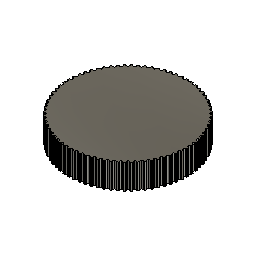
gear_76z (Autodesk Fusion 360 design; units mm, degrees)
Autodesk Fusion 360 part; units mm, degrees
sketch "Sketch1" plane through (0, 0, 0) normal (0, 0, 1) x (1, 0, 0) in component "gt2 pulley"
  circle A0 centre (0, 0) radius 24.1916 construction
  circle A1 centre (0, 0) radius 23.1876 construction
  line L0 (0, 0) -> (0, 24.1916) construction
  line L1 (0, 0) -> (0.9997, 24.1709) construction
  line L2 (0, 0) -> (1.4051, 24.1507) construction
  circle A2 centre (0, 0) radius 23.9376 construction
  arc A3 (0.395, 23.8007) -> (0.4708, 23.5042) centre (1.3904, 23.8971) ccw
  circle A4 centre (0, 0) radius 23.7876 construction
  arc A5 (0.2472, 23.9363) -> (0, 23.9376) centre (0, 0) ccw
  arc A6 (0.395, 23.8007) -> (0.2472, 23.9363) centre (0.2457, 23.7863) ccw
  arc A7 (0.4708, 23.5042) -> (0.9582, 23.1677) centre (0.9812, 23.7223) ccw
  arc A8 (0, 23.9376) -> (-0.2472, 23.9363) centre (0, 0) ccw
  arc A9 (-0.2472, 23.9363) -> (-0.395, 23.8007) centre (-0.2457, 23.7863) ccw
  arc A10 (-0.4708, 23.5042) -> (-0.395, 23.8007) centre (-1.3904, 23.8971) ccw
  arc A11 (-0.958, 23.1678) -> (-0.4708, 23.5042) centre (-0.9812, 23.7223) ccw
  arc A12 (0.9582, 23.1677) -> (-0.9582, 23.1677) centre (0, 0) ccw
  point P0 (1.3904, 23.8971)
  point P1 (0, 23.9376)
  dimension "d18" = 48.3831
  dimension "d19" = 2.368
  dimension "d22" = 1.004
  dimension "d24" = 0.75
  dimension "d26" = 1
  dimension "d27" = 0.15
  dimension "d28" = 0.15
  dimension "d47" = 0.555
  dimension "d52" = 3.812
  constraint coincident A0.centre A1.centre
  constraint coincident A0 L0.end
  constraint vertical L0
  constraint coincident A0 L1.end
  constraint coincident A0 L2.end
  constraint concentric A1 A2
  constraint coincident A1 A7.end
  constraint coincident L1 A7.end
  constraint coincident A2 P0
  constraint coincident L2 P0
  constraint coincident P0 A3.centre
  constraint coincident A2 P1
  constraint coincident L0 P1
  constraint concentric A2 A4
  constraint coincident P1 A5.end
  constraint coincident A4 A6.centre
  constraint coincident A3.start A6.start
  constraint tangent A3 A6
  constraint tangent A3 A7
  constraint symmetric L0 A7.end A12.end
  constraint symmetric L0 A3.start A9.end
  constraint symmetric L0 A3.end A10.start
  constraint symmetric L0 A3 A10
  constraint symmetric L0 A5.start A8.end
  constraint symmetric L0 P1 A5.end
  constraint symmetric L0 A5 A8
  constraint symmetric L0 A6 A9
  constraint symmetric L0 A7 A11
  constraint coincident A1 A11.start
  constraint tangent A1 A7
  constraint coincident L1 A7.centre
  measures "d18" diameter of A0
  measures "d19" angle of L0 L1
  measures "d22" distance of A0 A1
  measures "d24" distance of A1 A2
  measures "d26" radius of A3
  measures "d27" distance of A2 A4
  measures "d28" radius of A6
  measures "d47" radius of A7
extrude "Extrude1" add sketch "Sketch1" along normal blind 10 makes body 1
pattern_circular "C-Pattern1" count 76 over 360 about axis through (0, 0, 1.75) along (0, 0, 1) of bodies 1 makes body 2 at (-1.171, 23.158, 3.3333) makes body 3 at (-3.9214, 22.8536, 6.6667) makes body 4 at (-6.4117, 22.2835, 6.6667) makes body 5 at (-6.8201, 22.1619, 3.3333) makes body 6 at (-9.992, 20.9242, 6.6667) makes body 7 at (-10.3748, 20.7371, 3.3333) makes body 8 at (-13.2997, 18.9942, 6.6667) makes body 9 at (-14.3259, 18.2327, 6.6667) makes body 10 at (-16.2446, 16.5461, 6.6667) makes body 11 at (-16.546, 16.2448, 3.3333) makes body 12 at (-17.831, 14.8229, 3.3333) makes body 13 at (-19.4698, 12.5932, 6.6667) makes body 14 at (-20.737, 10.375, 6.6667) makes body 15 at (-20.9241, 9.9921, 3.3333) makes body 16 at (-22.1618, 6.8203, 6.6667) makes body 17 at (-22.2834, 6.4118, 3.3333) makes body 18 at (-22.7368, 4.5498, 3.3333) makes body 19 at (-23.1169, 1.8088, 6.6667) makes body 20 at (-23.1756, -0.7452, 6.6667) makes body 21 at (-23.158, -1.171, 3.3333) makes body 22 at (-22.8536, -3.9214, 6.6667) makes body 23 at (-22.6494, -4.9667, 3.3333) makes body 24 at (-21.6779, -8.2299, 6.6667) makes body 25 at (-21.523, -8.6269, 3.3333) makes body 26 at (-20.7371, -10.3748, 3.3333) makes body 27 at (-18.9942, -13.2997, 6.6667) makes body 28 at (-18.2327, -14.3259, 6.6667) makes body 29 at (-16.5461, -16.2446, 6.6667) makes body 30 at (-16.2448, -16.546, 3.3333) makes body 31 at (-14.8229, -17.831, 3.3333) makes body 32 at (-13.2999, -18.9941, 3.3333) makes body 33 at (-10.375, -20.737, 6.6667) makes body 34 at (-9.2168, -21.2771, 6.6667) makes body 35 at (-6.8203, -22.1618, 6.6667) makes body 36 at (-6.4118, -22.2834, 3.3333) makes body 37 at (-4.5498, -22.7368, 3.3333) makes body 38 at (-1.8088, -23.1169, 6.6667) makes body 39 at (0.7452, -23.1756, 6.6667) makes body 40 at (2.4448, -23.0583, 6.6667) makes body 41 at (3.9214, -22.8536, 6.6667) makes body 42 at (6.4117, -22.2835, 6.6667) makes body 43 at (6.8201, -22.1619, 3.3333) makes body 44 at (9.992, -20.9242, 6.6667) makes body 45 at (10.3748, -20.7371, 3.3333) makes body 46 at (12.0518, -19.8095, 3.3333) makes body 47 at (14.3259, -18.2327, 6.6667) makes body 48 at (15.148, -17.5557, 3.3333) makes body 49 at (16.546, -16.2448, 3.3333) makes body 50 at (17.831, -14.8229, 3.3333) makes body 51 at (18.9941, -13.2999, 6.6667) makes body 52 at (20.737, -10.375, 6.6667) makes body 53 at (20.9241, -9.9921, 3.3333) makes body 54 at (22.1618, -6.8203, 6.6667) makes body 55 at (22.2834, -6.4118, 3.3333) makes body 56 at (22.7368, -4.5498, 3.3333) makes body 57 at (23.158, -1.1712, 6.6667) makes body 58 at (23.1756, 0.7452, 6.6667) makes body 59 at (23.158, 1.171, 3.3333) makes body 60 at (22.8536, 3.9214, 6.6667) makes body 61 at (22.6494, 4.9667, 3.3333) makes body 62 at (21.6779, 8.2299, 6.6667) makes body 63 at (21.523, 8.6269, 3.3333) makes body 64 at (20.7371, 10.3748, 3.3333) makes body 65 at (19.8095, 12.0518, 3.3333) makes body 66 at (18.7466, 13.6465, 3.3333) makes body 67 at (16.9874, 15.7826, 6.6667) makes body 68 at (16.2448, 16.546, 3.3333) makes body 69 at (14.8229, 17.831, 3.3333) makes body 70 at (13.2999, 18.9941, 3.3333) makes body 71 at (10.375, 20.737, 6.6667) makes body 72 at (9.9921, 20.9241, 3.3333) makes body 73 at (6.8203, 22.1618, 6.6667) makes body 74 at (5.589, 22.5039, 6.6667) makes body 75 at (3.0795, 22.9821, 6.6667) makes body 76 at (2.6567, 23.0349, 3.3333)
sketch "Sketch2" plane through (0, 0, 10) normal (0, 0, 1) x (-1, 0, 0)
  arc A0 (-4.3071, -23.4111) -> (-4.1836, -23.5691) centre (-4.1575, -23.4214) ccw
  arc A1 (-4.1836, -23.5691) -> (-3.696, -23.6505) centre (0, 0) ccw
  arc A2 (-3.696, -23.6505) -> (-3.5278, -23.5411) centre (-3.6727, -23.5023) ccw
  arc A3 (-3.4043, -23.2611) -> (-3.5278, -23.5411) centre (-2.5619, -23.8001) ccw
  arc A4 (-2.8683, -23.0095) -> (-3.4043, -23.2611) centre (-2.9368, -23.5602) ccw
  arc A5 (-4.7584, -22.694) -> (-2.8683, -23.0095) centre (0, 0) ccw
  arc A6 (-4.333, -23.1061) -> (-4.7584, -22.694) centre (-4.8723, -23.2372) ccw
  arc A7 (-4.3071, -23.4111) -> (-4.333, -23.1061) centre (-5.3047, -23.3424) ccw
  circle A8 centre (0, 0) radius 23.1876
  constraint coincident A1.centre A5.centre
extrude "Extrude2" add sketch "Sketch2" against normal blind 10 contours A5 A8 bodies 1 2 3 4 5 6 7 8 9 10 11 12 13 14 15 16 17 18 19 20 21 22 23 24 25 26 27 28 29 30 31 32 33 34 35 36 37 38 39 40 41 42 43 44 45 46 47 48 49 50 51 52 53 54 55 56 57 58 59 60 61 62 63 64 65 66 67 68 69 70 71 72 73 74 75 76
extrude "Extrude4" [suppressed] in component "gt2 pulley"
pattern_circular "C-Pattern7" [suppressed] in component "gt2 pulley"
extrude "Extrude3" [suppressed] in component "gt2 pulley"
pattern_circular "C-Pattern6" [suppressed] in component "gt2 pulley"
extrude "Extrude2'" [suppressed] in component "gt2 pulley"
pattern_circular "C-Pattern5" [suppressed] in component "gt2 pulley"
extrude "Extrude1'" [suppressed] in component "gt2 pulley"
pattern_circular "C-Pattern4" [suppressed] in component "gt2 pulley"
pattern_circular "C-Pattern3" [suppressed] in component "gt2 pulley"
pattern_circular "C-Pattern2" [suppressed] in component "gt2 pulley"
pattern_circular "C-Pattern1'" [suppressed] in component "gt2 pulley"
copy_body "Body->Comp1" [suppressed] in component "Component"
copy_body "Body->Comp2" [suppressed] in component "Component'"
copy_body "Body->Comp3" [suppressed] in component "Component''"
copy_body "Body->Comp4" [suppressed] in component "Component'''"
copy_body "Body->Comp5" [suppressed] in component "Component''''"
copy_body "Body->Comp6" [suppressed] in component "Component'''''"
copy_body "Body->Comp7" [suppressed] in component "Component''''''"
copy_body "Body->Comp8" [suppressed] in component "Component'''''''"
copy_body "Body->Comp9" [suppressed] in component "Component''''''''"
copy_body "Body->Comp10" [suppressed] in component "Component'''''''''"
copy_body "Body->Comp11" [suppressed] in component "Component''''''''''"
copy_body "Body->Comp12" [suppressed] in component "Component'''''''''''"
copy_body "Body->Comp13" [suppressed] in component "Component''''''''''''"
copy_body "Body->Comp14" [suppressed] in component "Component'''''''''''''"
copy_body "Body->Comp15" [suppressed] in component "Component''''''''''''''"
copy_body "Body->Comp16" [suppressed] in component "Component'''''''''''''''"
copy_body "Body->Comp17" [suppressed] in component "Component''''''''''''''''"
copy_body "Body->Comp18" [suppressed] in component "Component'''''''''''''''''"
copy_body "Body->Comp19" [suppressed] in component "Component''''''''''''''''''"
copy_body "Body->Comp20" [suppressed] in component "Component'''''''''''''''''''"
component "gt2 pulley" placed x (1, 0, 0) y (0, 1, 0) z (0, 0, 1) at (0, 0, 0)
equation "NumTeeth = 76" comment "min 20"
equation "ToothPitch = 2 mm"
equation "PullyDia = NumTeeth * ToothPitch / PI"
equation "ToothAng = ( ( 360 / NumTeeth ) * 1 deg )"
equation "TransOffsetAngle = ToothAng * 0.2"
equation "Sholulder_Radius = 0.15 mm"
equation "Root_Radius = 0.555 mm"
equation "TransRadius = 1 mm"
equation "ToolHeight = 0.75 mm"
equation "PLD = 0.254 mm"
equation "d18 = PullyDia"
equation "d19 = ToothAng / 2"
equation "d22 = PLD + ToolHeight"
equation "d24 = ToolHeight"
equation "d26 = TransRadius"
equation "d27 = Sholulder_Radius"
equation "d31 = NumTeeth"
equation "d33 = NumTeeth"
equation "d35 = NumTeeth"
equation "d37 = NumTeeth"
equation "d41 = NumTeeth"
equation "d45 = NumTeeth"
equation "d47 = Root_Radius"
equation "d50 = NumTeeth"
